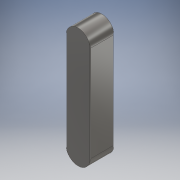
# Autodesk Inventor part: PulleyKey
Saved by Autodesk Inventor 2018 (Build 220112000, 112)
## iProperties
Created: 2018-05-29
Part Number: PulleyKey
Material: Steel, Alloy
Document SubType Name: Modeling
Designer: P136265
Density: 7.73 g/cm^3
Appearance: Semi-Polished
Author: P136265
Autodesk Inventor part; units mm, degrees
ref_plane "YZ Plane" through (0, 0, 0) normal (1, 0, 0) x (0, 1, 0)
ref_plane "XZ Plane" through (0, 0, 0) normal (0, 1, 0) x (-1, 0, 0)
ref_plane "XY Plane" through (0, 0, 0) normal (0, 0, 1) x (1, 0, 0)
sketch "Sketch1" plane through (0, 0, 0) normal (0, 0, 1) x (1, 0, 0)
  line L0 (-2, -2) -> (2, -2)
  line L1 (2, -2) -> (2, 2)
  line L2 (2, 2) -> (-2, 2)
  line L3 (-2, 2) -> (-2, -2)
  line L4 (-2, -2) -> (2, 2) construction
  line L5 (2, -2) -> (-2, 2) construction
  point P0 (0, 0)
  dimension "d0" = 4
  dimension "d1" = 4
  constraints: 12 end point, 2 midpoint, 2 parallel, 1 horizontal, 1 perpendicular
  measures "d0" distance of L2.end L1.end
  measures "d1" distance of L1.end L0.end
extrude "Extrusion1" add sketch "Sketch1" along normal mid plane 20
fillet "Fillet1" radius 2 4 edges at (2, 0, 10) (-2, 0, 10) (2, 0, -10) (-2, 0, -10)
fillet "Fillet1" radius 0.15 4 edges at (2, 2, 0) (-2, 2, 0) (2, -2, 0) (-2, -2, 0)
body "Solid1"
